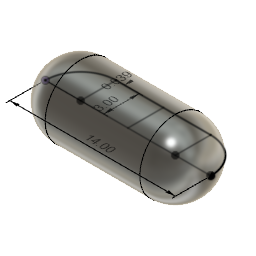
MUD 6 inch Tank v3 (Autodesk Fusion 360 design; units mm, degrees)
Autodesk Fusion 360 part; units mm, degrees
sketch "Sketch1" plane through (0, 0, 0) normal (0, 0, 1) x (1, 0, 0)
sketch "Sketch2" plane through (0, 0, 0) normal (0, 0, 1) x (1, 0, 0)
  line L0 (0, 0) -> (355.6, 0)
  line L1 (279.4, 76.2) -> (76.2, 76.2)
  arc A0 (76.2, 76.2) -> (0, 0) centre (76.2, 0) ccw
  line L2 (177.8, 76.2) -> (177.8, 0)
  arc A1 (355.6, 0) -> (279.4, 76.2) centre (279.4, 0) ccw
  arc A2 (354.6, 0) -> (279.4, 75.2) centre (279.4, 0) ccw
  line L3 (279.4, 75.2) -> (76.2, 75.2)
  arc A3 (76.2, 75.2) -> (1, 0) centre (76.2, 0) ccw
  line L4 (76.2, 0) -> (76.2, 76.2)
  line L5 (279.4, 0) -> (279.4, 76.2)
  dimension "d1" = 355.6
  dimension "d4" = 76.2
  dimension "d5" = -1
  constraint horizontal L0
  constraint horizontal L1
  constraint coincident L0.start A0.end
  constraint coincident L0 A0.centre
  constraint tangent L1 A0
  constraint midpoint L0 L2.end
  constraint symmetric L0.start L2 L0.end
  constraint symmetric A0 L2 A1
  constraint symmetric L1.end L2 L1.start
  constraint coincident L1 L2.start
  constraint coincident A0.centre A3.centre
  constraint coincident A1.centre A2.centre
  measures "d1" distance of L0.start L0.end
  measures "d4" distance of L0 L1
revolve "Revolve1" add sketch "Sketch2" angle 360 about axis through (0, 0, 0) along (1, 0, 0) contours L0 A0 A3 L4 makes body 1
revolve "Revolve2" add sketch "Sketch2" angle 360 about axis through (0, 0, 0) along (1, 0, 0) separate body contours L0 A3 L4 | L0 L2 L3 L4 | L0 L2 L3 L5 | L0 A2 L5 makes body 2
revolve "Revolve3" add sketch "Sketch2" angle 360 about axis through (0, 0, 0) along (1, 0, 0) separate body contours L0 A1 A2 L5 makes body 3
revolve "Revolve4" add sketch "Sketch2" angle 360 about axis through (0, 0, 0) along (1, 0, 0) separate body contours L1 L2 L3 L4 | L1 L2 L3 L5 makes body 4
copy_body "Body->Comp1" bodies 1 removing the originals makes body 5 in component "Component"
copy_body "Body->Comp2" bodies 3 removing the originals makes body 6 in component "Component'"
copy_body "Body->Comp3" bodies 4 removing the originals makes body 7 in component "Component''"
component "Component" placed x (1, 0, 0) y (0, 1, 0) z (0, 0, 1) at (0, 0, 0)
component "Component'" placed x (1, 0, 0) y (0, 1, 0) z (0, 0, 1) at (0, 0, 0)
component "Component''" placed x (1, 0, 0) y (0, 1, 0) z (0, 0, 1) at (0, 0, 0)
hidden bodies 2
